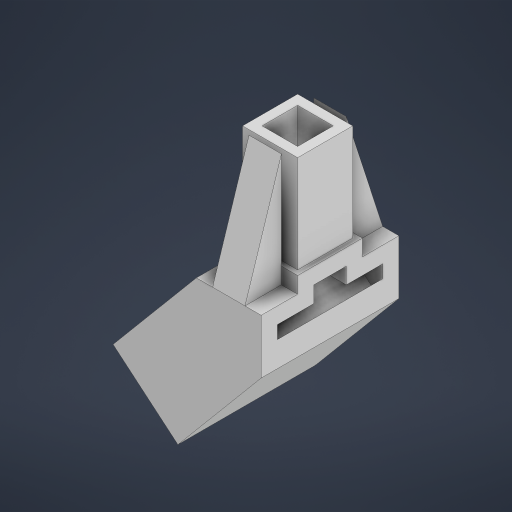
# Autodesk Inventor part: motor_holder
Saved by Autodesk Inventor 2024 (Build 280153000, 153)
## iProperties
Created: 2023-09-26
Part Number: motor_holder
Material: Типовые
Document SubType Name: Modeling
Designer: user
Density: 1 g/cm^3
Appearance: По умолчанию
Author: user
Autodesk Inventor part; units mm, degrees
ref_plane "YZ Plane" through (0, 0, 0) normal (1, 0, 0) x (0, 1, 0)
ref_plane "XZ Plane" through (0, 0, 0) normal (0, 1, 0) x (-1, 0, 0)
ref_plane "XY Plane" through (0, 0, 0) normal (0, 0, 1) x (1, 0, 0)
sketch "Эскиз1" plane through (0, 0, 0) normal (0, 0, 1) x (1, 0, 0)
  line L0 (0, 0) -> (20, 0) construction
  line L1 (20, 0) -> (20, 20) construction
  line L2 (20, 20) -> (0, 20) construction
  line L3 (0, 20) -> (0, 0) construction
  line L4 (1.5, 18.5) -> (18.5, 18.5)
  line L5 (18.5, 18.5) -> (18.5, 1.5)
  line L6 (18.5, 1.5) -> (1.5, 1.5)
  line L7 (1.5, 1.5) -> (1.5, 18.5)
  line L8 (15.5, 15.5) -> (4.5, 15.5)
  line L9 (4.5, 15.5) -> (4.5, 4.5)
  line L10 (4.5, 4.5) -> (15.5, 4.5)
  line L11 (15.5, 4.5) -> (15.5, 15.5)
  dimension "d0" = 20
  dimension "d1" = 20
  dimension "d2" = 1.5
  dimension "d3" = 3
  constraints: 24 end point, 6 parallel, 3 perpendicular, 1 horizontal, 6 other
  measures "d0" distance of L1.end L2.end
  measures "d1" distance of L0.end L1.end
  measures "d2" distance between parallel lines of L2 L4
  measures "d3" distance between parallel lines of L4 L8
extrude "Выдавливание1" add sketch "Эскиз1" along normal blind 30
sketch "Эскиз2" plane through (0, 0, 0) normal (0, 0, -1) x (-1, 0, 0)
  line L0 (-18.5, 18.5) -> (-1.5, 18.5) construction
  line L1 (-1.5, 18.5) -> (-1.5, 1.5) construction
  line L2 (-1.5, 1.5) -> (-18.5, 1.5) construction
  line L3 (-18.5, 1.5) -> (-18.5, 18.5) construction
  line L4 (0, 20) -> (-20, 20)
  line L5 (-20, 20) -> (-20, 0)
  line L6 (-20, 0) -> (0, 0)
  line L7 (0, 0) -> (0, 20)
  point P0 (0, 0)
  dimension "d6" = 1.5
  constraints: 8 end point, 3 other
  measures "d6" distance between parallel lines of L0 L4
extrude "Выдавливание2" add sketch "Эскиз2" along normal blind 5
ref_plane "РабПлоскость1" through (1.5, 10, 30) normal (0, -1, 0) x (1, 0, 0)
sketch "Эскиз3" plane through (1.5, 10, 30) normal (0, -1, 0) x (1, 0, 0)
  line L0 (-1.5, -35) -> (18.5, -35) projected
  line L1 (-1.5, -35) -> (18.5, -51.782)
  line L2 (18.5, -51.782) -> (18.5, -35)
  point P0 (-1.5, -30)
  dimension "d9" = 40
  constraints: 4 end point, 1 vertical
  measures "d9" angle of L0 L1
extrude "Выдавливание3" add sketch "Эскиз3" along normal mid plane 42.5
sketch "Эскиз4" plane through (20, -11.25, -21.782) normal (-0.6427876, 0, -0.7660444) x (-0.7660444, 0, 0.6427876)
  line L0 (0, 42.5) -> (0, 0) projected
  line L1 (26.1081, 0) -> (0, 0) projected
  line L2 (26.1081, 11.25) -> (26.1081, 0) projected
  line L3 (26.1081, 11.25) -> (26.1081, 31.25) projected
  line L4 (26.1081, 42.5) -> (26.1081, 31.25) projected
  line L5 (0, 42.5) -> (26.1081, 42.5) projected
extrude "Выдавливание4" add sketch "Эскиз4" along normal blind 40
ref_plane "РабПлоскость2" through (10, 1.5, 30) normal (-1, 0, 0) x (0, 0, 1)
sketch "Эскиз5" plane through (10, 1.5, 30) normal (-1, 0, 0) x (0, 0, 1)
  line L0 (-30, 18.5) -> (-35, 18.5) projected
  line L1 (-30, 18.5) -> (0, 18.5)
  line L2 (-35, 29.75) -> (-65.6418, 29.75) projected
  line L3 (0, 18.5) -> (-35, 29.75)
  line L4 (-35, 18.5) -> (-35, 29.75) projected
  point P0 (-30, -1.5)
  dimension "d14" = 30
  constraints: 4 end point, 1 horizontal
  measures "d14" distance of L0.start L1.end
extrude "Выдавливание5" add sketch "Эскиз5" along normal mid plane 10
mirror "Зеркальное отражение1" about plane through (1.5, 10, 30) normal (0, -1, 0) of "Выдавливание5"
sketch "Эскиз6" plane through (-5.7115, -11.25, -52.4238) normal (-0.6427876, 0, -0.7660444) x (-0.7660444, 0, 0.6427876)
  line L0 (26.1081, 42.5) -> (26.1081, 31.25) projected
  line L1 (26.1081, 36.5) -> (4, 36.5)
  line L2 (4, 36.5) -> (4, 6)
  line L3 (4, 6) -> (26.1081, 6)
  line L4 (26.1081, 6) -> (26.1081, 36.5)
  line L5 (0, 42.5) -> (0, 0) projected
  line L6 (0, 0) -> (26.1081, 0) projected
  point P0 (29.3221, 11.25)
  point P1 (26.1081, 21.25)
  point P2 (0, 21.25)
  point P3 (26.1081, 31.25)
  dimension "d18" = 6
  dimension "d19" = 4
  constraints: 8 end point, 2 midpoint, 2 parallel, 1 horizontal, 1 horizontal alignment, 1 perpendicular, 1 point on line
  measures "d18" distance from line of L6 L3.end
  measures "d19" distance between parallel lines of L5 L2
extrude "Выдавливание6" cut sketch "Эскиз6" against normal blind 36
shell "Оболочка1" thickness 5 removed faces 1 at (20, 13.3333, -16.188)
equation "\"d1\" = d0"
